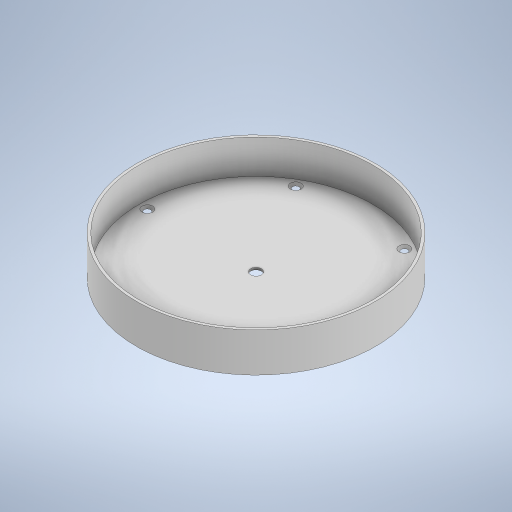
# Autodesk Inventor part: bowl
Saved by Autodesk Inventor 2023 (Build 270158000, 158)
## iProperties
Created: 2025-12-15
Part Number: bowl
Material: Generic
Document SubType Name: Modeling
Designer: Justin Pascual
Density: 1 g/cm^3
Appearance: Default
Author: Justin Pascual
Autodesk Inventor part; units mm, degrees
ref_plane "YZ Plane" through (0, 0, 0) normal (1, 0, 0) x (0, 1, 0)
ref_plane "XZ Plane" through (0, 0, 0) normal (0, 1, 0) x (-1, 0, 0)
ref_plane "XY Plane" through (0, 0, 0) normal (0, 0, 1) x (1, 0, 0)
sketch "Sketch1" plane through (0, 0, 0) normal (0, 1, 0) x (-1, 0, 0)
  circle A0 centre (0, 0) radius 139.7
  dimension "d0" = 279.4
  constraints: 1 centre point, 1 coincident
  measures "d0" diameter of A0
extrude "Extrusion1" add sketch "Sketch1" along normal blind 45.72
sketch "Sketch3" plane through (0, 45.72, 0) normal (0, 1, 0) x (1, 0, 0)
  circle A0 centre (0, 0) radius 136.652
  dimension "d7" = 273.304
  constraints: 1 centre point, 1 coincident
  measures "d7" diameter of A0
extrude "Extrusion3" cut sketch "Sketch3" against normal blind 39.878
sketch "Sketch4" plane through (0, 0, 0) normal (0, -1, 0) x (1, 0, 0)
  circle A0 centre (0, 0) radius 137.16
  dimension "d10" = 274.32
  constraints: 1 centre point, 1 coincident
  measures "d10" diameter of A0
extrude "Extrusion5" cut sketch "Sketch4" against normal blind 3.3782
sketch "Sketch5" plane through (0, 3.3782, 0) normal (0, -1, 0) x (1, 0, 0)
  circle A0 centre (0, 0) radius 115.8875
  circle A1 centre (0, 0) radius 113.3475
  dimension "d15" = 231.775
  dimension "d16" = 226.695
  constraints: 2 centre point, 2 coincident
  measures "d15" diameter of A0
  measures "d16" diameter of A1
extrude "Extrusion6" add sketch "Sketch5" along normal blind 5.4102
sketch "Sketch6" plane through (0, 5.842, 0) normal (0, 1, 0) x (1, 0, 0)
  circle A0 centre (0, 0) radius 6.35
  dimension "d19" = 12.7
  constraints: 1 centre point, 1 coincident
  measures "d19" diameter of A0
extrude "Extrusion7" cut sketch "Sketch6" against normal through all
sketch "Sketch7" plane through (0, 5.842, 0) normal (0, -1, 0) x (1, 0, 0)
  point P0 (0, 0)
  point P1 (127, 0)
  point P2 (63.5, 109.9852)
  point P3 (-63.5, 109.9852)
  point P4 (-127, 0)
  point P5 (-63.5, -109.9852)
  point P6 (63.5, -109.9852)
  dimension "d22" = 127
  dimension "d25" = 360
  constraints: 7 other
  measures "d22" distance of point (0, 0) point (127, 0)
hole "Hole1" at (127, 5.842, 0) at (63.5, 5.842, 109.9852) at (-63.5, 5.842, 109.9852) at (-127, 5.842, 0) at (-63.5, 5.842, -109.9852) at (63.5, 5.842, -109.9852) direction (0, -1, 0) diameter 6.604 end through all countersink diameter 12.5984 countersink angle 90 clearance for "Flat Head Machine Screw" size "M6" standard "Ansi Metric M Profile"
body "Solid1"
